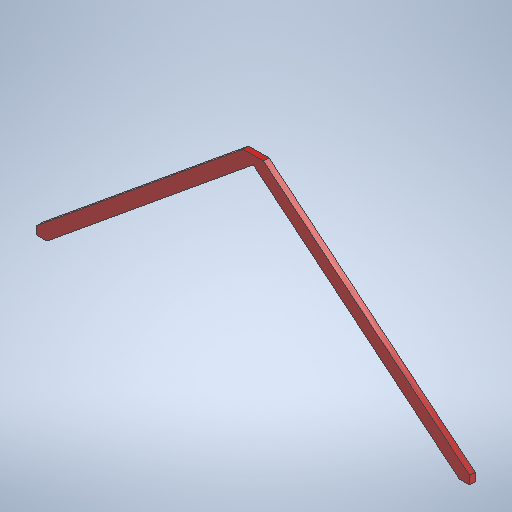
# Autodesk Inventor part: side1
Saved by Autodesk Inventor 2025.1 (Build 291241020, 241B)
## iProperties
Created: 2024-09-20
Part Number: side1
Material: Generic
Document SubType Name: Modeling
Designer: User
Density: 1 g/cm^3
Appearance: Default
Author: User
Autodesk Inventor part; units mm, degrees
ref_plane "YZ Plane" through (0, 0, 0) normal (1, 0, 0) x (0, 1, 0)
ref_plane "XZ Plane" through (0, 0, 0) normal (0, 1, 0) x (-1, 0, 0)
ref_plane "XY Plane" through (0, 0, 0) normal (0, 0, 1) x (1, 0, 0)
sketch "Sketch1" plane through (0, 0, 0) normal (0, 0, 1) x (1, 0, 0)
  line L0 (3048, 0) -> (0, 0) projected
  line L1 (38.1, 1219.2) -> (38.1, 0) projected
  line L2 (3048, 1219.2) -> (0, 1219.2) projected
  line L3 (3009.9, 1219.2) -> (3009.9, 0) projected
  line L4 (3009.9, 57.4978) -> (1594.0754, 1219.2)
  line L5 (1453.9246, 1219.2) -> (38.1, 57.4978)
  line L6 (108.1754, 0) -> (1524, 1161.7022)
  line L7 (1524, 1161.7022) -> (2939.8246, 0)
  line L8 (3009.9, 57.4978) -> (3009.9, 0)
  line L9 (2939.8246, 0) -> (3009.9, 0)
  line L10 (1594.0754, 1219.2) -> (1453.9246, 1219.2)
  line L11 (38.1, 57.4978) -> (38.1, 0)
  line L12 (38.1, 0) -> (108.1754, 0)
  constraints: 18 end point, 6 point on line, 3 collinear, 2 parallel, 2 perpendicular, 2 other
extrude "Extrusion1" add sketch "Sketch1" against normal blind 38.1 contours L0 L7 L6 L1 L5 L2 L4 L3
body "Solid1"
